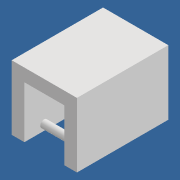
# Autodesk Inventor part: MotorHolder_X
Saved by Autodesk Inventor 2020 (Build 240168000, 168)
## iProperties
Created: 2019-12-21
Part Number: MotorHolder_X
Material: Generic
Document SubType Name: Modeling
Designer: Jack
Density: 1 g/cm^3
Appearance: Default
Author: Jack
Autodesk Inventor part; units mm, degrees
ref_plane "YZ Plane" through (0, 0, 0) normal (1, 0, 0) x (0, 1, 0)
ref_plane "XZ Plane" through (0, 0, 0) normal (0, 1, 0) x (-1, 0, 0)
ref_plane "XY Plane" through (0, 0, 0) normal (0, 0, 1) x (1, 0, 0)
sketch "Sketch1" plane through (0, 0, 0) normal (1, 0, 0) x (0, 1, 0)
  line L0 (-19.8, 28) -> (19.8, 28)
  line L1 (19.8, 28) -> (19.8, -28)
  line L2 (19.8, -28) -> (-19.8, -28)
  line L3 (-19.8, -28) -> (-19.8, 28)
  line L4 (-19.8, 28) -> (19.8, -28) construction
  line L5 (19.8, 28) -> (-19.8, -28) construction
  point P0 (0, 0)
  dimension "d0" = 39.6
  dimension "d1" = 56
  constraints: 12 end point, 2 midpoint, 2 parallel, 1 horizontal, 1 perpendicular
  measures "d0" distance of L1.end L2.end
  measures "d1" distance of L0.end L1.end
extrude "Extrusion1" add sketch "Sketch1" along normal blind 40
sketch "Sketch2" plane through (0, -19.8, 28) normal (0, 0, 1) x (1, 0, 0)
  line L0 (7.8, 0) -> (32.2, 0)
  line L1 (32.2, 0) -> (32.2, 31.8)
  line L2 (32.2, 31.8) -> (7.8, 31.8)
  line L3 (7.8, 31.8) -> (7.8, 0)
  line L4 (0, 0) -> (40, 0) projected
  line L5 (40, 39.6) -> (40, 0) projected
  dimension "d4" = 24.4
  dimension "d5" = 31.8
  dimension "d6" = 7.8
  constraints: 8 end point, 2 parallel, 1 horizontal, 1 perpendicular, 1 point on line
  measures "d4" distance of L2.end L1.end
  measures "d5" distance of L1.end L0.end
  measures "d6" distance between parallel lines of L5 L1
extrude "Extrusion2" cut sketch "Sketch2" against normal blind 64
sketch "Sketch3" plane through (32.2, -19.8, 28) normal (-1, 0, 0) x (0, 0, 1)
  circle A0 centre (-12, 3.8502) radius 2.3
  circle A1 centre (-28, 3.8502) radius 2.3
  line L0 (0, 31.8) -> (0, 0) projected
  point P0 (-28, 19.8)
  dimension "d9" = 4.6
  dimension "d10" = 4.6
  dimension "d11" = 16
  dimension "d12" = 12
  constraints: 2 centre point, 1 horizontal alignment
  measures "d9" diameter of A0
  measures "d10" diameter of A1
  measures "d11" distance of A1.centre A0.centre
  measures "d12" distance from line of L0 A0.centre
extrude "Extrusion3" add sketch "Sketch3" along normal blind 26
sketch "Sketch4" plane through (7.8, -19.8, 28) normal (1, 0, 0) x (0, 0, -1)
  line L0 (56, 0) -> (0, 0) projected
  line L1 (56, 0) -> (32, 0)
  line L2 (32, 0) -> (32, 8)
  line L3 (32, 8) -> (56, 8)
  line L4 (56, 8) -> (56, 0)
  point P0 (28, 19.8)
  point P1 (32, 0)
  dimension "d15" = 24
  dimension "d16" = 8
  constraints: 8 end point, 2 parallel, 1 horizontal, 1 perpendicular
  measures "d15" distance of L2.end L3.end
  measures "d16" distance of L1.end L2.end
extrude "Extrusion4" add sketch "Sketch4" along normal blind 26
body "Solid1"
